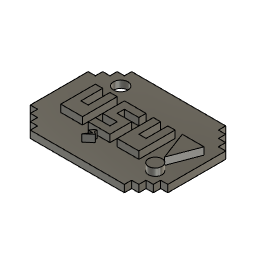
brelocUSU (Autodesk Fusion 360 design; units mm, degrees)
Autodesk Fusion 360 part; units mm, degrees
sketch "Sketch1" plane through (0, 0, 0) normal (0, 0, 1) x (1, 0, 0)
  line L0 (-25, 0) -> (-15, 0)
  line L1 (-15, 0) -> (-15, 5)
  line L2 (-15, 5) -> (-10, 5)
  line L3 (-10, 5) -> (-10, 10)
  line L4 (-10, 10) -> (-5, 10)
  line L5 (-5, 10) -> (-5, 15)
  line L6 (-5, 15) -> (-1.7883, 15)
  line L7 (-1.7883, 15) -> (0, 15)
  line L8 (0, 15) -> (0, 55)
  line L9 (0, 55) -> (-5, 55)
  line L10 (-5, 55) -> (-5, 60)
  line L11 (-5, 60) -> (-10, 60)
  line L12 (-10, 60) -> (-10, 65)
  line L13 (-10, 65) -> (-15, 65)
  line L14 (-15, 65) -> (-15, 70)
  line L15 (-15, 70) -> (-80, 70)
  line L16 (-80, 70) -> (-80, 65)
  line L17 (-80, 65) -> (-85, 65)
  line L18 (-85, 65) -> (-85, 60)
  line L19 (-85, 60) -> (-90, 60)
  line L20 (-90, 60) -> (-90, 55)
  line L21 (-90, 55) -> (-95, 55)
  line L22 (-95, 55) -> (-95, 15)
  line L23 (-95, 15) -> (-90, 15)
  line L24 (-90, 15) -> (-90, 10)
  line L25 (-90, 10) -> (-85, 10)
  line L26 (-85, 10) -> (-85, 5)
  line L27 (-85, 5) -> (-80, 5)
  line L28 (-80, 5) -> (-80, 0)
  line L29 (-80, 0) -> (-25, 0)
  constraint horizontal L0
  constraint perpendicular L0 L1
  constraint perpendicular L1 L2
  constraint perpendicular L2 L3
  constraint perpendicular L3 L4
  constraint perpendicular L4 L5
  constraint perpendicular L5 L6
  constraint perpendicular L5 L7
  constraint perpendicular L6 L8
  constraint perpendicular L8 L9
  constraint perpendicular L6 L10
  constraint perpendicular L10 L11
  constraint perpendicular L11 L12
  constraint perpendicular L10 L13
  constraint perpendicular L13 L14
  constraint perpendicular L14 L15
  constraint perpendicular L15 L16
  constraint perpendicular L16 L17
  constraint perpendicular L17 L18
  constraint perpendicular L16 L19
  constraint perpendicular L17 L20
  constraint perpendicular L20 L21
  constraint perpendicular L9 L22
  constraint perpendicular L22 L23
  constraint perpendicular L23 L24
  constraint perpendicular L24 L25
  constraint perpendicular L25 L26
  constraint perpendicular L24 L27
  constraint perpendicular L17 L28
  constraint perpendicular L28 L29
extrude "Extrude1" add sketch "Sketch1" along normal blind 5
hole "Hole1" at (-75.2055, 57.6429, 5) direction (0, 0, -1) diameter 10 depth 30 tip angle 118
sketch "Sketch2" plane through (0, 0, 5) normal (0, 0, 1) x (-1, 0, 0)
  circle A0 centre (75.2055, -57.6429) radius 5
  line L0 (80, 0) -> (15, 0)
  line L1 (15, 0) -> (15, -5)
  line L2 (15, -5) -> (10, -5)
  line L3 (10, -5) -> (10, -10)
  line L4 (10, -10) -> (5, -10)
  line L5 (5, -10) -> (5, -15)
  line L6 (5, -15) -> (0, -15)
  line L7 (0, -15) -> (0, -55)
  line L8 (0, -55) -> (5, -55)
  line L9 (5, -55) -> (5, -60)
  line L10 (5, -60) -> (10, -60)
  line L11 (10, -60) -> (10, -65)
  line L12 (10, -65) -> (15, -65)
  line L13 (15, -65) -> (15, -70)
  line L14 (15, -70) -> (80, -70)
  line L15 (80, -70) -> (80, -65)
  line L16 (80, -65) -> (85, -65)
  line L17 (85, -65) -> (85, -60)
  line L18 (85, -60) -> (90, -60)
  line L19 (90, -60) -> (90, -55)
  line L20 (90, -55) -> (95, -55)
  line L21 (95, -55) -> (95, -15)
  line L22 (95, -15) -> (90, -15)
  line L23 (90, -15) -> (90, -10)
  line L24 (90, -10) -> (85, -10)
  line L25 (85, -10) -> (85, -5)
  line L26 (85, -5) -> (80, -5)
  line L27 (80, -5) -> (80, 0)
  line L28 (80, -45) -> (80, -21.0556)
  line L29 (80, -21.0556) -> (65, -21.0556)
  line L30 (65, -21.0556) -> (65, -43.5828)
  line L31 (65, -43.5828) -> (65, -45)
  line L32 (65, -45) -> (70, -45)
  line L33 (70, -45) -> (70, -30)
  line L34 (70, -30) -> (75, -30)
  line L35 (75, -30) -> (75, -45)
  line L36 (75, -45) -> (80, -45)
  line L37 (60, -45) -> (45, -45)
  line L38 (45, -45) -> (45, -40)
  line L39 (45, -40) -> (55, -40)
  line L40 (55, -40) -> (55, -35)
  line L41 (55, -35) -> (45, -35)
  line L42 (45, -35) -> (45, -25)
  line L43 (45, -25) -> (45, -20)
  line L44 (45, -20) -> (60, -20)
  line L45 (60, -20) -> (60, -25)
  line L46 (60, -25) -> (50, -25)
  line L47 (50, -25) -> (50, -30)
  line L48 (50, -30) -> (60, -30)
  line L49 (60, -30) -> (60, -45)
  line L50 (40, -45) -> (40, -20)
  line L51 (40, -20) -> (25, -20)
  line L52 (25, -20) -> (25, -45)
  line L53 (25, -45) -> (30, -45)
  line L54 (30, -45) -> (30, -30)
  line L55 (30, -30) -> (35, -30)
  line L56 (35, -30) -> (35, -45)
  line L57 (35, -45) -> (40, -45)
  line L58 (20, -45) -> (5, -45)
  line L59 (5, -45) -> (12.5, -25.2503)
  line L60 (12.5, -25.2503) -> (20, -45)
  circle A1 centre (12.4062, -18.7252) radius 4.684
  line L61 (53.32, -17.4727) -> (55, -15)
  line L62 (55, -15) -> (51.9633, -15)
  line L63 (51.9633, -15) -> (55, -10.5305)
  line L64 (55, -10.5305) -> (50, -15)
  line L65 (50, -15) -> (51.9633, -16.3339)
  line L66 (51.9633, -16.3339) -> (51.9633, -18.151)
  line L67 (51.9633, -18.151) -> (53.32, -17.4727)
  constraint parallel L21 L28
  constraint perpendicular L28 L29
  constraint perpendicular L29 L30
  constraint perpendicular L31 L32
  constraint perpendicular L32 L33
  constraint perpendicular L33 L34
  constraint perpendicular L34 L35
  constraint perpendicular L28 L36
  constraint horizontal L37
  constraint perpendicular L37 L38
  constraint perpendicular L38 L39
  constraint perpendicular L37 L40
  constraint perpendicular L40 L41
  constraint perpendicular L41 L42
  constraint perpendicular L41 L43
  constraint perpendicular L43 L44
  constraint perpendicular L44 L45
  constraint perpendicular L45 L46
  constraint perpendicular L46 L47
  constraint perpendicular L47 L48
  constraint perpendicular L46 L49
  constraint parallel L38 L50
  constraint perpendicular L50 L51
  constraint perpendicular L51 L52
  constraint perpendicular L52 L53
  constraint perpendicular L53 L54
  constraint perpendicular L54 L55
  constraint perpendicular L55 L56
  constraint perpendicular L50 L57
  constraint perpendicular L54 L58
  constraint parallel L46 L62
  constraint parallel L61 L63
  constraint perpendicular L63 L65
extrude "Extrude2" add sketch "Sketch2" along normal blind 5 contours L28 L29 L30 L31 L32 L33 L34 L35 L36 | L37 L38 L39 L40 L41 L42 L43 L44 L45 L46 L47 L48 L49 | L50 L51 L52 L53 L54 L55 L56 L57 | L58 L59 L60 | A1 | L61 L62 L63 L64 L65 L66 L67
